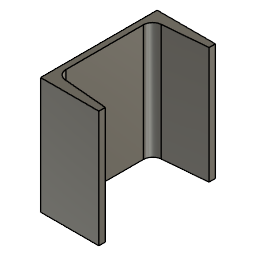
C-100×50×5×7.5 (Autodesk Fusion 360 design; units mm, degrees)
Autodesk Fusion 360 part; units mm, degrees
note: some values were not read from the file. Set by a fixed rule: which sketch regions a step uses.
sketch "スケッチ1" plane through (0, 0, 0) normal (0, 0, 1) x (1, 0, 0)
  line L0 (5, 83.2009) -> (5, 16.7991)
  line L1 (0, 100) -> (0, 0)
  line L2 (0, 0) -> (50, 0)
  line L3 (12.3028, 8.8296) -> (50, 5.5315)
  arc A0 (5, 16.7991) -> (12.3028, 8.8296) centre (13, 16.7991) ccw
  line L4 (50, 5.5315) -> (50, 0)
  line L5 (50, 94.4685) -> (12.3028, 91.1704)
  line L6 (0, 100) -> (50, 100)
  arc A1 (12.3028, 91.1704) -> (5, 83.2009) centre (13, 83.2009) ccw
  line L7 (50, 100) -> (50, 94.4685)
extrude "押し出し1" add sketch "スケッチ1" along normal blind 100
